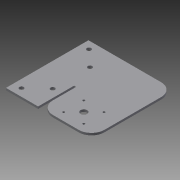
# Autodesk Inventor part: ARMS MOUNTING BRACKET
Saved by Autodesk Inventor 2015 (Build 190159000, 159)
## iProperties
Created: 2015-02-10
Part Number: ARMS MOUNTING BRACKET
Material: Generic
Document SubType Name: Modeling
Designer: chapale16
Density: 1 g/cm^3
Appearance: Default
Author: chapale16
Autodesk Inventor part; units mm, degrees
ref_plane "YZ Plane" through (0, 0, 0) normal (1, 0, 0) x (0, 1, 0)
ref_plane "XZ Plane" through (0, 0, 0) normal (0, 1, 0) x (-1, 0, 0)
ref_plane "XY Plane" through (0, 0, 0) normal (0, 0, 1) x (1, 0, 0)
sketch "Sketch1" plane through (0, 0, 0) normal (0, 1, 0) x (-1, 0, 0)
  line L0 (0, 0) -> (-127, 0)
  line L1 (-127, 0) -> (-127, -122.428)
  line L2 (-127, -122.428) -> (0, -122.428)
  line L3 (0, -122.428) -> (0, 0)
  line L4 (0, 0) -> (-47.752, 0)
  line L5 (-47.752, 0) -> (-47.752, -53.34)
  line L6 (-47.752, -53.34) -> (0, -53.34)
  line L7 (0, -53.34) -> (0, 0)
  line L8 (-127, -122.428) -> (-50.8, -122.428)
  line L9 (-50.8, -122.428) -> (-50.8, 0)
  line L10 (-50.8, 0) -> (-127, 0)
  line L11 (-127, 0) -> (-127, -122.428)
  line L12 (-47.752, -53.34) -> (-50.8, -53.34)
  line L13 (-50.8, -53.34) -> (-50.8, 0)
  line L14 (-50.8, 0) -> (-47.752, 0)
  line L15 (-47.752, 0) -> (-47.752, -53.34)
  circle A0 centre (-11.938, -11.176) radius 3.175
  circle A1 centre (-35.814, -33.528) radius 3.175
  circle A2 centre (-11.938, -111.252) radius 3.175
  circle A3 centre (-35.814, -88.9) radius 3.175
  circle A4 centre (-73.914, -11.684) radius 1.5875
  circle A5 centre (-73.914, -41.656) radius 1.5875
  circle A6 centre (-103.886, -41.656) radius 1.5875
  circle A7 centre (-103.886, -11.684) radius 1.5875
  circle A8 centre (-88.9, -26.67) radius 4.953
  dimension "d0" = 127
  dimension "d1" = 122.428
  dimension "d2" = 47.752
  dimension "d3" = 53.34
  dimension "d4" = 76.2
  dimension "d5" = 11.176
  dimension "d6" = 22.352
  dimension "d7" = 38.1
  dimension "d8" = 14.986
  dimension "d9" = 14.986
  dimension "d10" = 14.986
  dimension "d11" = 14.986
  dimension "d12" = 6.35
  dimension "d13" = 6.35
  dimension "d14" = 6.35
  dimension "d15" = 6.35
  dimension "d16" = 3.175
  dimension "d17" = 3.175
  dimension "d18" = 3.175
  dimension "d19" = 3.175
  dimension "d20" = 9.906
  dimension "d21" = 11.176
  dimension "d22" = 11.938
  dimension "d23" = 23.876
  dimension "d24" = 22.352
  dimension "d25" = 11.938
  dimension "d26" = 11.938
  dimension "d27" = 23.876
  constraints: 32 end point, 9 centre point, 9 coincident, 8 parallel, 4 horizontal, 4 perpendicular, 1 point on line
  measures "d0" distance of L2.end L1.end
  measures "d1" distance of L1.end L0.end
  measures "d2" distance of L6.end L5.end
  measures "d3" distance of L5.end L4.end
  measures "d4" distance of L10.end L9.end
  measures "d5" distance from line of L2 point (-11.938, -111.252)
  measures "d6" vertical distance of point (-11.938, -111.252) point (-35.814, -88.9)
  measures "d7" distance from line of L13 point (-88.9, -26.67)
  measures "d8" horizontal distance of point (-73.914, -11.684) point (-88.9, -26.67)
  measures "d9" horizontal distance of point (-73.914, -11.684) point (-88.9, -26.67)
  measures "d10" horizontal distance of point (-88.9, -26.67) point (-103.886, -11.684)
  measures "d11" horizontal distance of point (-73.914, -41.656) point (-88.9, -26.67)
  measures "d12" diameter of A0
  measures "d13" diameter of A1
  measures "d14" diameter of A2
  measures "d15" diameter of A3
  measures "d16" diameter of A4
  measures "d17" diameter of A5
  measures "d18" diameter of A6
  measures "d19" diameter of A7
  measures "d20" diameter of A8
  measures "d21" distance from line of L0 A0.centre
  measures "d22" distance from line of L3 point (-11.938, -11.176)
  measures "d23" horizontal distance of A0.centre A1.centre
  measures "d24" vertical distance of A0.centre A1.centre
  measures "d25" distance from line of L15 A1.centre
  measures "d26" distance from line of L3 point (-11.938, -111.252)
  measures "d27" horizontal distance of A2.centre point (-35.814, -88.9)
extrude "Extrusion1" add sketch "Sketch1" along normal blind 3.175 contours L3 L6 L5 L0 | L3 L2 L9 L12 L6 | L9 L2 L1 L0
fillet "Fillet1" radius 19.05 3 edges at (127, 1.5875, 0) (50.8, 1.5875, 0) (127, 1.5875, -122.428)
body "Solid1"
